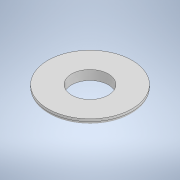
# Autodesk Inventor part: wheel_chain_guide_holes
Saved by Autodesk Inventor 2021 (Build 250183000, 183)
## iProperties
Created: 2021-08-01
Part Number: wheel_chain_guide_holes
Material: Generic
Document SubType Name: Modeling
Designer: Mateusz
Density: 1 g/cm^3
Appearance: Default
Author: Mateusz
Autodesk Inventor part; units mm, degrees
ref_plane "YZ Plane" through (0, 0, 0) normal (1, 0, 0) x (0, 1, 0)
ref_plane "XZ Plane" through (0, 0, 0) normal (0, 1, 0) x (-1, 0, 0)
ref_plane "XY Plane" through (0, 0, 0) normal (0, 0, 1) x (1, 0, 0)
sketch "Sketch1" plane through (0, 0, 0) normal (0, 1, 0) x (-1, 0, 0)
  circle A0 centre (0, 0) radius 52
  circle A1 centre (0, 0) radius 22.75
  circle A2 centre (0, 0) radius 27.5
  dimension "d2" = 45.5
  dimension "d4" = 55
  constraints: 3 centre point, 2 coincident
  measures "d2" diameter of A1
  measures "d4" diameter of A2
extrude "Extrusion1" add sketch "Sketch1" against normal blind 4.75 contours A2
extrude "Extrusion2" add sketch "Sketch1" along normal blind 7 contours A0 | A2
fillet "Fillet1" radius 4 1 edges at (52, 0, 0)
body "Solid1"
